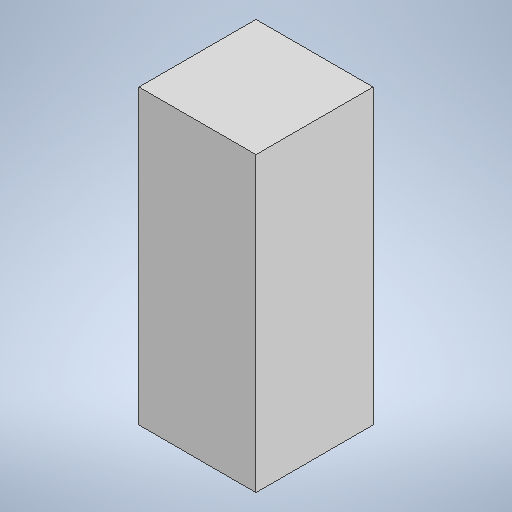
# Autodesk Inventor part: BX11111
Saved by Autodesk Inventor 2027 (Build 310192060, 192F)
## iProperties
Created: 2026-08-01
Part Number: BX11111
Material: Generic
Document SubType Name: Modeling
Designer: TiffanyHayden
Density: 1 g/cm^3
Appearance: Default
DEPTH: 5
LENGTH: 2
WIDTH: 2
Author: TiffanyHayden
Autodesk Inventor part; units mm, degrees
ref_plane "YZ Plane" through (0, 0, 0) normal (1, 0, 0) x (0, 1, 0)
ref_plane "XZ Plane" through (0, 0, 0) normal (0, 1, 0) x (-1, 0, 0)
ref_plane "XY Plane" through (0, 0, 0) normal (0, 0, 1) x (1, 0, 0)
sketch "Sketch1" plane through (0, 0, 0) normal (0, 1, 0) x (-1, 0, 0)
  line L0 (-25.4, 25.4) -> (25.4, 25.4)
  line L1 (25.4, 25.4) -> (25.4, -25.4)
  line L2 (25.4, -25.4) -> (-25.4, -25.4)
  line L3 (-25.4, -25.4) -> (-25.4, 25.4)
  line L4 (-25.4, 25.4) -> (25.4, -25.4) construction
  line L5 (25.4, 25.4) -> (-25.4, -25.4) construction
  point P0 (0, 0)
  dimension "d0" = 50.8
  dimension "d1" = 50.8
  constraints: 12 end point, 2 midpoint, 2 parallel, 1 horizontal, 1 perpendicular
  measures "d0" distance of L1.end L2.end
  measures "d1" distance of L0.end L1.end
extrude "Extrusion1" add sketch "Sketch1" along normal blind 127
body "Solid1"
